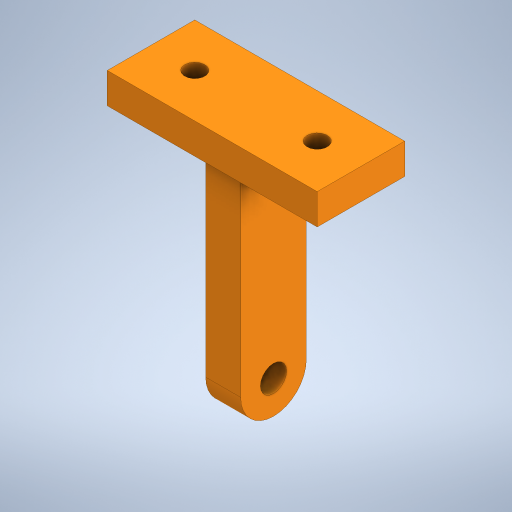
# Autodesk Inventor part: RouleauMount
Saved by Autodesk Inventor 2023 (Build 270158000, 158)
## iProperties
Created: 2022-09-08
Part Number: RouleauMount
Material: Generic
Document SubType Name: Modeling
Designer: Nathann
Density: 1 g/cm^3
Appearance: Orange
Author: Nathann
Autodesk Inventor part; units mm, degrees
ref_plane "YZ Plane" through (0, 0, 0) normal (1, 0, 0) x (0, 1, 0)
ref_plane "XZ Plane" through (0, 0, 0) normal (0, 1, 0) x (-1, 0, 0)
ref_plane "XY Plane" through (0, 0, 0) normal (0, 0, 1) x (1, 0, 0)
sketch "Sketch1" plane through (0, 0, 0) normal (1, 0, 0) x (0, 1, 0)
  circle A0 centre (0, 0) radius 3
  circle A1 centre (0, 0) radius 7.5
  line L0 (0, 7.5) -> (45, 7.5)
  line L1 (45, 7.5) -> (45, -7.5)
  line L2 (45, -7.5) -> (0, -7.5)
  dimension "d0" = 6
  dimension "d1" = 15
  dimension "d2" = 45
  constraints: 6 end point, 2 centre point, 2 coincident, 2 point on circle, 1 horizontal, 1 perpendicular, 1 tangent
  measures "d0" diameter of A0
  measures "d1" diameter of A1
  measures "d2" distance from line of point (0, 0) L1
extrude "Extrusion1" add sketch "Sketch1" along normal blind 8
sketch "Sketch2" plane through (0, 0, 0) normal (-1, 0, 0) x (0, 0, 1)
  line L0 (-10, 45) -> (10, 45)
  line L1 (10, 45) -> (10, 52)
  line L2 (10, 52) -> (-10, 52)
  line L3 (-10, 52) -> (-10, 45)
  line L4 (7.5, 45) -> (7.5, 0) projected
  line L5 (-7.5, 45) -> (7.5, 45) projected
  point P0 (0, 0)
  dimension "d5" = 20
  dimension "d6" = 2.5
  dimension "d7" = 0
  dimension "d8" = 7
  constraints: 8 end point, 2 parallel, 1 horizontal, 1 perpendicular
  measures "d5" distance of L1.end L2.end
  measures "d6" distance between parallel lines of L1 L4
  measures "d7" distance between parallel lines of L5 L0
  measures "d8" distance between parallel lines of L0 L2
extrude "Extrusion2" add sketch "Sketch2" along normal blind 20 and the other way blind 28
sketch "Sketch3" plane through (-20, 45, 10) normal (0, -1, 0) x (1, 0, 0)
  circle A0 centre (38, -10) radius 2.3
  circle A1 centre (10, -10) radius 2.3
  line L0 (48, 0) -> (0, 0) projected
  line L1 (48, 0) -> (48, -20) projected
  line L2 (0, -20) -> (0, 0) projected
  point P0 (20, -10)
  dimension "d13" = 10
  dimension "d14" = 10
  dimension "d15" = 4.6
  dimension "d16" = 4.6
  dimension "d17" = 10
  dimension "d18" = 10
  constraints: 2 centre point
  measures "d13" distance from line of L0 A1.centre
  measures "d14" distance from line of L0 A0.centre
  measures "d15" diameter of A0
  measures "d16" diameter of A1
  measures "d17" distance from line of L1 A0.centre
  measures "d18" distance from line of L2 A1.centre
extrude "Extrusion3" cut sketch "Sketch3" against normal mid plane 20
equation "\"d14\" = d13"
equation "\"d15\" = d16"
equation "\"d17\" = d14"
equation "\"d18\" = d13"
body "Solid1"
